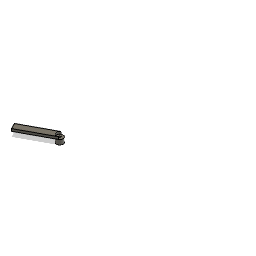
Quick Remoal Lock (Autodesk Fusion 360 design; units mm, degrees)
Autodesk Fusion 360 part; units mm, degrees
sketch "Sketch1" plane through (-3.8469, 25.504, -6.2551) normal (0, 1, 0) x (-0.866025, 0, 0.5)
  line L0 (-70.5762, 109.5047) -> (-57.8146, 87.2541)
  line L1 (-57.8146, 87.2541) -> (-52.8571, 90.0974)
  line L2 (-52.8571, 90.0974) -> (-77.6585, 133.3403)
  arc A0 (77.7753, 132.8951) -> (-77.6585, 133.3403) centre (-0.3236, -0.2219) ccw
  line L3 (77.7753, 132.8951) -> (52.7383, 89.8153)
  line L4 (52.7383, 89.8153) -> (57.6877, 86.9578)
  line L5 (57.6877, 86.9578) -> (70.5177, 109.0338)
  arc A1 (70.5177, 109.0338) -> (75.0016, 116.7489) centre (71.1126, 113.8485) ccw
  line L6 (75.0016, 116.7489) -> (85.5254, 134.8567)
  arc A2 (85.5254, 134.8567) -> (67.303, 144.8399) centre (-0.3236, -0.2219) ccw
  arc A3 (67.303, 144.8399) -> (58.5412, 148.6109) centre (62.571, 145.9097) ccw
  arc A4 (58.5412, 148.6109) -> (-58.3308, 148.9472) centre (-0.3236, -0.2219) ccw
  arc A5 (-58.3308, 148.9472) -> (-67.1377, 145.2159) centre (-62.4162, 146.3307) ccw
  arc A6 (-67.1377, 145.2159) -> (-85.3973, 135.3463) centre (-0.3236, -0.2219) ccw
  line L7 (-85.3973, 135.3463) -> (-75.0157, 117.2454)
  arc A7 (-75.0157, 117.2454) -> (-70.5762, 109.5047) centre (-71.1434, 114.3228) ccw
  circle A8 centre (-71.1434, 114.3228) radius 2.413
  circle A9 centre (62.571, 145.9097) radius 2.413
  circle A10 centre (71.1126, 113.8485) radius 2.413
  circle A11 centre (-62.4162, 146.3307) radius 2.413
  line L8 (9.8635, 54.1416) -> (30.8082, 54.0816)
  line L9 (30.8082, 54.0816) -> (76.4164, 132.5572)
  arc A12 (76.4164, 132.5572) -> (-75.8952, 132.9935) centre (-0.1202, -0.1463) ccw
  line L10 (-75.8952, 132.9935) -> (-28.5496, 50.4433)
  line L11 (-28.5496, 50.4433) -> (7.6539, 50.3396)
  line L12 (7.6539, 50.3396) -> (9.8635, 54.1416)
  line L13 (27.0551, 70.999) -> (19.1357, 73.3288)
  line L14 (19.1357, 73.3288) -> (17.3103, 67.1242)
  arc A13 (17.3103, 67.1242) -> (-16.4749, 67.3937) centre (-0.1202, -0.1463) ccw
  line L15 (-16.4749, 67.3937) -> (-17.3301, 73.1405)
  line L16 (-17.3301, 73.1405) -> (-25.4952, 71.9255)
  line L17 (-25.4952, 71.9255) -> (-24.4586, 64.9591)
  arc A14 (-27.8836, 66.3841) -> (-24.4586, 64.9591) centre (-25.242, 67.9047) ccw
  line L18 (-27.8836, 66.3841) -> (-57.9427, 118.6031)
  spline S0 degree 3 poles (-57.3225, 122.405) (-57.6196, 122.1418) (-57.8624, 121.823) (-58.1694, 121.1976) (-58.2608, 120.9109) (-58.3091, 120.616) (-58.3583, 120.3152) (-58.3621, 120.006) (-58.2663, 119.3174) (-58.1377, 118.9419) (-57.9427, 118.6031) knots 0 0 0 0 0.099224 0.099224 0.174187 0.174187 0.174187 0.250654 0.250654 0.348375 0.348375 0.348375 0.348375
  spline S1 degree 3 poles (-56.8832, 122.8261) (-56.9082, 122.8002) (-56.9334, 122.7744) (-57.0429, 122.664) (-57.1159, 122.588) (-57.3225, 122.405) knots 0.501684 0.501684 0.501684 0.501684 0.51252 0.51252 0.548438 0.548438 0.548438 0.548438
  line L19 (-56.8832, 122.8261) -> (-51.8571, 121.6841)
  line L20 (-51.8571, 121.6841) -> (-50.0811, 129.5006)
  line L21 (-50.0811, 129.5006) -> (-55.1072, 130.6426)
  spline S2 degree 3 poles (-55.3214, 131.2122) (-55.3025, 131.1675) (-55.2841, 131.1225) (-55.2088, 130.934) (-55.1558, 130.789) (-55.1072, 130.6426) knots 0.287713 0.287713 0.287713 0.287713 0.302282 0.302282 0.348613 0.348613 0.348613 0.348613
  spline S3 degree 3 poles (-53.6938, 135.2061) (-53.7708, 135.1737) (-53.8463, 135.1383) (-54.2846, 134.9102) (-54.6101, 134.6457) (-55.0629, 134.0931) (-55.2197, 133.8299) (-55.3349, 133.5477) (-55.4086, 133.3672) (-55.4646, 133.1803) (-55.5629, 132.6852) (-55.5766, 132.37) (-55.5099, 131.769) (-55.4353, 131.4825) (-55.3214, 131.2122) knots 0 0 0 0 0.020872 0.020872 0.12391 0.12391 0.200135 0.200135 0.200135 0.248905 0.248905 0.326939 0.326939 0.400269 0.400269 0.400269 0.400269
  spline S4 degree 3 poles (54.2606, 134.9843) (45.747, 138.6041) (36.907, 141.3564) (18.8431, 145.0616) (9.5982, 146.0141) (0.3472, 146.0359) (-8.9263, 146.0577) (-18.1821, 145.1489) (-27.282, 143.3208) (-36.3378, 141.5016) (-45.1853, 138.7825) (-53.6938, 135.2061) knots 0.297101 0.297101 0.297101 0.297101 3.064946 3.064946 5.832791 5.832791 5.832791 8.607361 8.607361 8.607361 11.368481 11.368481 11.368481 11.368481
  spline S5 degree 3 poles (55.8594, 130.9553) (56.0605, 131.4139) (56.1456, 131.92) (56.0829, 132.7203) (56.0139, 133.019) (55.9016, 133.3023) (55.8307, 133.4812) (55.7432, 133.6525) (55.476, 134.0729) (55.2715, 134.3076) (54.804, 134.7031) (54.5415, 134.8649) (54.2606, 134.9843) knots 0 0 0 0 0.125191 0.125191 0.201434 0.201434 0.201434 0.249555 0.249555 0.326549 0.326549 0.402867 0.402867 0.402867 0.402867
  spline S6 degree 3 poles (55.6365, 130.3872) (55.694, 130.5526) (55.7638, 130.7374) (55.8594, 130.9553) knots 0.128256 0.128256 0.128256 0.128256 0.181735 0.181735 0.181735 0.181735
  line L22 (55.6365, 130.3872) -> (50.5682, 129.2891)
  line L23 (50.5682, 129.2891) -> (52.277, 121.4021)
  line L24 (52.277, 121.4021) -> (57.3453, 122.5002)
  spline S7 degree 3 poles (57.7833, 122.0753) (57.6431, 122.201) (57.5766, 122.2664) (57.4475, 122.3944) (57.396, 122.4469) (57.3453, 122.5002) knots 0.206215 0.206215 0.206215 0.206215 0.329636 0.329636 0.413668 0.413668 0.413668 0.413668
  spline S8 degree 3 poles (58.3817, 118.2699) (58.5817, 118.6127) (58.7128, 118.9913) (58.8091, 119.6814) (58.8064, 119.9824) (58.7601, 120.2776) (58.7129, 120.5787) (58.6199, 120.8736) (58.3138, 121.4978) (58.0744, 121.8144) (57.7833, 122.0753) knots 0 0 0 0 0.099224 0.099224 0.174189 0.174189 0.174189 0.250656 0.250656 0.348379 0.348379 0.348379 0.348379
  line L25 (58.3817, 118.2699) -> (28.024, 66.224)
  arc A15 (25.2071, 64.7172) -> (28.024, 66.224) centre (25.3912, 67.7597) ccw
  line L26 (25.2071, 64.7172) -> (27.0551, 70.999)
  circle A16 centre (-62.2526, 127.6747) radius 4.508
  circle A17 centre (-19.942, 60.736) radius 4.508
  circle A18 centre (-55.8217, 106.3902) radius 2.413
  circle A19 centre (-41.3576, 80.9732) radius 2.413
  circle A20 centre (-29.1627, 60.7624) radius 2.413
  circle A21 centre (0.052, 59.9375) radius 8.382
  circle A22 centre (29.2708, 60.595) radius 2.413
  circle A23 centre (41.5813, 80.7356) radius 2.413
  circle A24 centre (56.1908, 106.0693) radius 2.413
  circle A25 centre (62.7375, 127.3166) radius 4.508
  circle A26 centre (20.0529, 60.6214) radius 4.508
  circle A27 centre (62.571, 145.9097) radius 1.7
  circle A28 centre (-62.4162, 146.3307) radius 1.7
  circle A29 centre (-62.4162, 146.3307) radius 4.8514
  line L27 (61.7951, 141.0609) -> (-62.4325, 141.4794)
  line L28 (62.5874, 150.7611) -> (-62.3998, 151.1821)
  circle A30 centre (62.571, 145.9097) radius 4.8514
  dimension "d5" = 3.4
  dimension "d6" = 3.4
  constraint concentric A3 A27
  constraint concentric A5 A28
  constraint concentric A28 A29
  constraint coincident A0 L27.start
  constraint coincident A29 L27.end
  constraint tangent A29 L27
  constraint coincident A29 L28.end
  constraint coincident A5 L28.end
  constraint tangent A29 L28
  constraint concentric A27 A30
  constraint coincident A2.end A30
  constraint tangent L27 A30
  constraint tangent L28 A30
  constraint coincident A3 L28.start
  measures "d5" diameter of A27
  measures "d6" diameter of A28
extrude "Extrude1" add sketch "Sketch1" along normal blind 7.112 contours A0 A3 A30 | A9
sketch "Sketch2" plane through (0, 32.616, 0) normal (0, 1, 0) x (-1, 0, 0)
  circle A0 centre (-14.9198, 151.3919) radius 1.7
  arc A1 (-13.4265, 146.7761) -> (-15.3006, 146.5555) centre (-14.9198, 151.3919) ccw
  arc A2 (-13.4265, 146.7761) -> (-15.3006, 146.5555) centre (3.6777, -6.6091) ccw
  line L0 (-12.6201, 147.1203) -> (32.4352, 171.3767)
  line L1 (32.4352, 171.3767) -> (27.8357, 179.92)
  line L2 (27.8357, 179.92) -> (-17.2196, 155.6636)
  constraint coincident A1 L0.start
  constraint perpendicular L0 L1
  constraint coincident A1 L2.end
  constraint perpendicular L1 L2
  constraint tangent A1 L0
  constraint tangent A1 L2
extrude "Extrude2" add sketch "Sketch2" along normal blind 3.556 contours A1 L0 L1 L2
